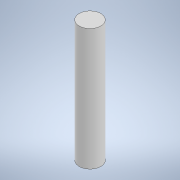
# Autodesk Inventor part: 3DPipeBoquilla0.4
Saved by Autodesk Inventor 2022 (Build 260153000, 153)
## iProperties
Created: 2022-04-01
Part Number: 3DPipeBoquilla0.4
Material: Genérico
Document SubType Name: Modeling
Designer: anuar
Density: 1 g/cm^3
Appearance: Valor por defecto
Author: anuar
Autodesk Inventor part; units mm, degrees
ref_plane "YZ Plane" through (0, 0, 0) normal (1, 0, 0) x (0, 1, 0)
ref_plane "XZ Plane" through (0, 0, 0) normal (0, 1, 0) x (-1, 0, 0)
ref_plane "XY Plane" through (0, 0, 0) normal (0, 0, 1) x (1, 0, 0)
sketch "Boceto1" plane through (0, 0, 0) normal (0, 0, 1) x (1, 0, 0)
  line L0 (0.99, 0) -> (0.99, 11.1361)
  line L1 (0.99, 11.1361) -> (0, 11.1361)
  line L2 (0, 11.1361) -> (0, 0)
  line L3 (0, 0) -> (0.99, 0)
  dimension "d9" = 0.99
  constraints: 8 end point, 1 horizontal
  measures "d9" distance between parallel lines of L2 L0
revolve "Revolución1" add sketch "Boceto1" angle 360 about axis through (0, 11.1361, 0) along (0, -1, 0)
equation "\"d9\" = 0.5 * Do"
equation "\"Dc\" = 0.4"
equation "\"Lc\" = 0.62"
equation "\"Ln\" = 10.06"
equation "\"Do\" = 1.98"
equation "\"alfa\" = 60deg"
